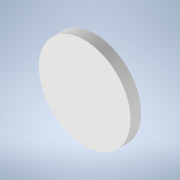
# Autodesk Inventor part: Circulo_Inferior
Saved by Autodesk Inventor 2022 (Build 260153000, 153)
## iProperties
Created: 2021-09-21
Part Number: Circulo_Inferior
Material: Generic
Document SubType Name: Modeling
Designer: Administrador
Density: 1 g/cm^3
Appearance: Default
Author: Administrador
Autodesk Inventor part; units mm, degrees
ref_plane "YZ Plane" through (0, 0, 0) normal (1, 0, 0) x (0, 1, 0)
ref_plane "XZ Plane" through (0, 0, 0) normal (0, 1, 0) x (-1, 0, 0)
ref_plane "XY Plane" through (0, 0, 0) normal (0, 0, 1) x (1, 0, 0)
sketch "Sketch3" plane through (0, 0, 0) normal (0, 0, 1) x (1, 0, 0)
  circle A0 centre (0, 0) radius 10.4
  circle A1 centre (-4.7579, 6.3065) radius 0.975 projected
  circle A2 centre (4.7579, -6.3065) radius 0.975 projected
  circle A3 centre (-4.7579, 6.3065) radius 0.975
  circle A4 centre (4.7579, -6.3065) radius 0.975
  dimension "d0" = 20.8
  constraints: 3 centre point, 3 coincident, 2 concentric
  measures "d0" diameter of A0
extrude "Extrusion1" add sketch "Sketch3" along normal blind 2.4
sketch "Sketch4" plane through (0, 0, 0) normal (0, 0, -1) x (-1, 0, 0)
  circle A0 centre (0, 0) radius 4.35
  circle A1 centre (0, 0) radius 2.7
  dimension "d3" = 8.7
  dimension "d4" = 5.4
  constraints: 2 centre point, 2 coincident
  measures "d3" diameter of A0
  measures "d4" diameter of A1
extrude "Extrusion2" add sketch "Sketch4" along normal blind 2.4 contours A0 | A1
sketch "Sketch5" plane through (0, 0, -2.4) normal (0, 0, -1) x (-1, 0, 0)
  circle A0 centre (0, 0) radius 2.7
  dimension "d7" = 5.4
  constraints: 1 centre point, 1 coincident
  measures "d7" diameter of A0
extrude "Extrusion3" cut sketch "Sketch5" against normal blind 2.8
sketch "Sketch6" plane through (0, 0, 2.4) normal (0, 0, 1) x (1, 0, 0)
  circle A0 centre (0, 0) radius 2.85
  dimension "d10" = 5.7
  constraints: 1 centre point, 1 coincident
  measures "d10" diameter of A0
extrude "Extrusion4" cut sketch "Sketch6" against normal blind 1
sketch "Sketch7" plane through (0, 0, 1.4) normal (0, 0, 1) x (1, 0, 0)
  circle A0 centre (0, 0) radius 4.35 projected
  circle A1 centre (0, 0) radius 1.5
  dimension "d13" = 3
  constraints: 1 centre point, 1 coincident
  measures "d13" diameter of A1
extrude "Extrusion5" cut sketch "Sketch7" against normal through all contours A1
body "Solid1"
